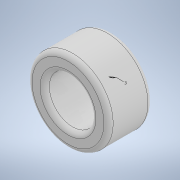
# Autodesk Inventor part: rulmanyatagıipt
Saved by Autodesk Inventor 2020 (Build 240168000, 168)
## iProperties
Created: 2021-12-23
Part Number: rulmanyatagıipt
Material: Generic
Document SubType Name: Modeling
Designer: Umur Batuhan Özmen
Density: 1 g/cm^3
Appearance: Default
Author: Umur Batuhan Özmen
Autodesk Inventor part; units mm, degrees
ref_plane "YZ Plane" through (0, 0, 0) normal (1, 0, 0) x (0, 1, 0)
ref_plane "XZ Plane" through (0, 0, 0) normal (0, 1, 0) x (-1, 0, 0)
ref_plane "XY Plane" through (0, 0, 0) normal (0, 0, 1) x (1, 0, 0)
sketch "Sketch1" plane through (0, 0, 0) normal (0, 0, 1) x (1, 0, 0)
  circle A0 centre (0, 0) radius 10.05
  circle A1 centre (0, 0) radius 17.5
  dimension "d0" = 20.1
  dimension "d2" = 35
  constraints: 2 centre point, 2 coincident
  measures "d0" diameter of A0
  measures "d2" diameter of A1
extrude "Extrusion1" add sketch "Sketch1" against normal blind 19
sketch "Sketch2" plane through (0, 0, -19) normal (0, 0, -1) x (-1, 0, 0)
  circle A0 centre (0, 0) radius 10.05
  circle A1 centre (0, 0) radius 1.5
  dimension "d7" = 3
  constraints: 2 centre point, 2 coincident
  measures "d7" diameter of A1
extrude "Extrusion2" add sketch "Sketch2" against normal blind 3.5 contours A0 | A1
extrude "Extrusion3" cut sketch "Sketch2" against normal blind 3.5 contours A1
fillet "Fillet1" radius 2 1 edges at (-10.05, 0, 0)
fillet "Fillet2" radius 2 2 edges at (-17.5, 0, 0) (-17.5, 0, -19)
body "Solid1"
